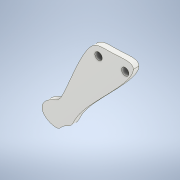
# Autodesk Inventor part: Component30
Saved by Autodesk Inventor 2022 (Build 260153000, 153)
## iProperties
Created: 2022-01-29
Part Number: Component30
Material: Generic
Document SubType Name: Modeling
Designer: Administrator
Density: 1 g/cm^3
Appearance: Default
Title: Component30
Author: Administrator
Autodesk Inventor part; units mm, degrees
ref_plane "YZ Plane" through (0, 0, 0) normal (1, 0, 0) x (0, 1, 0)
ref_plane "XZ Plane" through (0, 0, 0) normal (0, 1, 0) x (-1, 0, 0)
ref_plane "XY Plane" through (0, 0, 0) normal (0, 0, 1) x (1, 0, 0)
sketch "Sketch2" plane through (0, 0, 0) normal (0, 0, 1) x (1, 0, 0)
  circle A0 centre (36.813, 28.0831) radius 3.25
  circle A1 centre (13.1848, 28.1259) radius 3.25
  spline S0 degree 5 poles (43.9223, 33.3904) (43.9223, 32.6786) (43.6712, 31.0826) (42.5368, 28.1871) (39.5902, 23.4748) (33.9312, 16.4912) (26.912, 8.8275) (19.2371, 0.8905) (11.6322, -6.9152) (4.7567, -14.2245) (-0.8739, -20.7306) (-4.974, -26.214) (-7.5622, -30.5639) (-9.0655, -33.8105) (-10.1993, -36.1104) (-11.6156, -37.7157) (-13.8879, -38.9453) (-16.6359, -40.1682) (-18.914, -41.6516) (-20.303, -43.3862) (-21.6416, -44.9396) (-24.0907, -45.7235) (-27.9531, -45.2951) (-32.4081, -43.4963) (-36.1285, -40.4171) (-37.7893, -36.405) (-36.3197, -32.0603) (-32.4921, -28.2349) (-27.9757, -25.5678) (-24.3916, -24.1813) (-22.1898, -23.0927) (-20.0112, -20.2258) (-17.4318, -15.0348) (-14.1899, -7.5785) (-10.3602, 1.4345) (-6.1427, 10.9959) (-1.8208, 19.9727) (2.3604, 27.3683) (6.2662, 32.5181) (10.0023, 35.3872) (13.864, 36.5013) (18.1742, 36.635) (23.1446, 36.5599) (28.7474, 36.7975) (34.5304, 37.2954) (39.6672, 37.4461) (42.5461, 36.6969) (43.6712, 35.3534) (43.9223, 34.1022) (43.9223, 33.3904) knots 0 0 0 0 0 0 0.022222 0.044444 0.066667 0.088889 0.111111 0.133333 0.155556 0.177778 0.2 0.222222 0.244444 0.266667 0.288889 0.311111 0.333333 0.355556 0.377778 0.4 0.422222 0.444444 0.466667 0.488889 0.511111 0.533333 0.555556 0.577778 0.6 0.622222 0.644444 0.666667 0.688889 0.711111 0.733333 0.755556 0.777778 0.8 0.822222 0.844444 0.866667 0.888889 0.911111 0.933333 0.955556 0.977778 1 1 1 1 1 1 weights 1 1 1 1 1 1 1 1 1 1 1 1 1 1 1 1 1 1 1 1 1 1 1 1 1 1 1 1 1 1 1 1 1 1 1 1 1 1 1 1 1 1 1 1 1 1 1 1 1 1
  point P0 (0, 0)
  point P1 (-101.3685, 95.1139)
  dimension "d2" = 6.5
  constraints: 2 centre point, 1 equal radius, 1 other
  measures "d2" diameter of A1
extrude "Extrusion1" add sketch "Sketch2" along normal blind 5
equation "\"d2\" = R"
equation "\"d0\" = thickness"
equation "\"R\" = 6.5"
equation "\"thickness\" = 5"
equation "\"width\" = 6.5"
equation "\"R1\" = 9"
body "Solid1"
